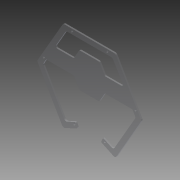
# Autodesk Inventor part: Top Plat
Saved by Autodesk Inventor 2015 (Build 190159000, 159)
## iProperties
Created: 2016-10-14
Part Number: Top Plat
Material: Polycarbonate, Clear
Document SubType Name: Modeling
Designer: James Yelland
Density: 1.2 g/cm^3
Appearance: Polycarbonate - Clear
Author: James Yelland
Autodesk Inventor part; units mm, degrees
ref_plane "YZ Plane" through (0, 0, 0) normal (1, 0, 0) x (0, 1, 0)
ref_plane "XZ Plane" through (0, 0, 0) normal (0, 1, 0) x (-1, 0, 0)
ref_plane "XY Plane" through (0, 0, 0) normal (0, 0, 1) x (1, 0, 0)
sketch "Sketch1" plane through (0, 0, 0) normal (0, 1, 0) x (-1, 0, 0)
  circle A0 centre (30.6147, -73.9104) radius 1.6
  circle A1 centre (-30.6147, -73.9104) radius 1.6
  circle A2 centre (30.6147, -73.9104) radius 1.6
  circle A3 centre (-30.6147, -73.9104) radius 1.6
  line L0 (103.5566, -2.5) -> (54.8095, -86.9325)
  line L1 (-54.8095, -86.9325) -> (-103.5566, -2.5)
  line L2 (-103.5566, 2.5) -> (-53.9434, 88.4327)
  line L3 (-49.6132, 90.9327) -> (49.6132, 90.9327)
  line L4 (53.9434, 88.4327) -> (103.5566, 2.5)
  arc A4 (48.3297, -88.9468) -> (54.8095, -86.9325) centre (50.4794, -84.4325) ccw
  arc A5 (-54.8095, -86.9325) -> (-48.3297, -88.9468) centre (-50.4794, -84.4325) ccw
  arc A6 (-103.5566, 2.5) -> (-103.5566, -2.5) centre (-99.2265, 0) ccw
  arc A7 (-49.6132, 90.9327) -> (-53.9434, 88.4327) centre (-49.6132, 85.9327) ccw
  arc A8 (53.9434, 88.4327) -> (49.6132, 90.9327) centre (49.6132, 85.9327) ccw
  arc A9 (103.5566, -2.5) -> (103.5566, 2.5) centre (99.2265, 0) ccw
  arc A10 (-43.8396, 80.9325) -> (-48.1698, 78.4325) centre (-43.8396, 75.9325) ccw
  arc A11 (-92.0094, 2.5) -> (-92.0094, -2.5) centre (-87.6793, 0) ccw
  line L5 (32.3518, -70.2624) -> (44.2883, -75.9464)
  arc A12 (44.2883, -75.9464) -> (50.7681, -73.9321) centre (46.4379, -71.4321) ccw
  line L6 (32.3518, -70.2624) -> (29.6432, -68.9726)
  line L7 (26.9776, -69.9184) -> (24.398, -75.3356)
  arc A13 (29.6432, -68.9726) -> (26.9776, -69.9184) centre (28.7834, -70.7783) ccw
  arc A14 (24.398, -75.3356) -> (25.3439, -78.0012) centre (26.2038, -76.1955) ccw
  circle A15 centre (-30.6147, -73.9104) radius 1.6
  circle A16 centre (-30.6147, -73.9104) radius 1.6
  line L8 (-32.3518, -70.2624) -> (-44.2883, -75.9464)
  arc A17 (-50.7681, -73.9321) -> (-44.2883, -75.9464) centre (-46.4379, -71.4321) ccw
  line L9 (-32.3518, -70.2624) -> (-29.6432, -68.9726)
  line L10 (-26.9776, -69.9184) -> (-24.398, -75.3356)
  arc A18 (-26.9776, -69.9184) -> (-29.6432, -68.9726) centre (-28.7834, -70.7783) ccw
  arc A19 (-25.3439, -78.0012) -> (-24.398, -75.3356) centre (-26.2038, -76.1955) ccw
  line L11 (48.3297, -88.9468) -> (25.3439, -78.0012)
  line L12 (-25.3439, -78.0012) -> (-48.3297, -88.9468)
  arc A20 (48.1698, 78.4325) -> (43.8396, 80.9325) centre (43.8396, 75.9325) ccw
  arc A21 (92.0094, -2.5) -> (92.0094, 2.5) centre (87.6793, 0) ccw
  circle A22 centre (35.5991, 85.9437) radius 1.6
  circle A23 centre (-35.5945, 85.9327) radius 1.6
  circle A24 centre (92.2171, 12.1406) radius 1.6
  circle A25 centre (-92.2171, 12.1406) radius 1.6
  line L13 (-18.2679, -8.3495) -> (18.2679, -8.3495)
  line L14 (-92.0094, -2.5) -> (-50.7681, -73.9321)
  line L15 (50.7681, -73.9321) -> (92.0094, -2.5)
  line L16 (59.1367, 11.2915) -> (33.0718, 11.2915)
  line L17 (59.1367, 11.2915) -> (85.2016, 11.2915)
  line L18 (53.75, 35.5415) -> (53.75, 17.0415)
  line L19 (53.75, 17.0415) -> (41.25, 17.0415)
  line L20 (41.25, 17.0415) -> (41.25, 35.5415)
  line L21 (41.25, 35.5415) -> (53.75, 35.5415)
  line L22 (53.75, 35.5415) -> (41.25, 17.0415) construction
  line L23 (53.75, 17.0415) -> (41.25, 35.5415) construction
  line L24 (71.75, 35.5415) -> (71.75, 17.0415)
  line L25 (71.75, 17.0415) -> (59.25, 17.0415)
  line L26 (59.25, 17.0415) -> (59.25, 35.5415)
  line L27 (59.25, 35.5415) -> (71.75, 35.5415)
  line L28 (71.75, 35.5415) -> (59.25, 17.0415) construction
  line L29 (71.75, 17.0415) -> (59.25, 35.5415) construction
  line L30 (92.0094, 2.5) -> (87.7997, 9.7915)
  line L31 (30.4737, 9.7915) -> (20.866, -6.8495)
  line L32 (-59.1367, 11.2915) -> (-33.0718, 11.2915)
  line L33 (-59.1367, 11.2915) -> (-85.2016, 11.2915)
  line L34 (-92.0094, 2.5) -> (-87.7997, 9.7915)
  line L35 (-30.4737, 9.7915) -> (-20.866, -6.8495)
  arc A26 (87.7997, 9.7915) -> (85.2016, 11.2915) centre (85.2016, 8.2915) ccw
  arc A27 (33.0718, 11.2915) -> (30.4737, 9.7915) centre (33.0718, 8.2915) ccw
  arc A28 (64.417, 41.2915) -> (67.0151, 45.7915) centre (64.417, 44.2915) ccw
  arc A29 (30.4737, 42.7915) -> (33.0718, 41.2915) centre (33.0718, 44.2915) ccw
  arc A30 (18.2679, -8.3495) -> (20.866, -6.8495) centre (18.2679, -5.3495) ccw
  arc A31 (-20.866, -6.8495) -> (-18.2679, -8.3495) centre (-18.2679, -5.3495) ccw
  arc A32 (-30.4737, 9.7915) -> (-33.0718, 11.2915) centre (-33.0718, 8.2915) ccw
  arc A33 (-33.0718, 41.2915) -> (-30.4737, 42.7915) centre (-33.0718, 44.2915) ccw
  arc A34 (-18.2679, 60.9325) -> (-20.866, 59.4325) centre (-18.2679, 57.9325) ccw
  arc A35 (20.866, 59.4325) -> (18.2679, 60.9325) centre (18.2679, 57.9325) ccw
  arc A36 (-67.0151, 45.7915) -> (-64.417, 41.2915) centre (-64.417, 44.2915) ccw
  arc A37 (-85.2016, 11.2915) -> (-87.7997, 9.7915) centre (-85.2016, 8.2915) ccw
  line L36 (43.8396, 80.9325) -> (-43.8396, 80.9325)
  line L37 (-48.1698, 78.4325) -> (-67.0151, 45.7915)
  line L38 (-64.417, 41.2915) -> (-33.0718, 41.2915)
  line L39 (-30.4737, 42.7915) -> (-20.866, 59.4325)
  line L40 (-18.2679, 60.9325) -> (18.2679, 60.9325)
  line L41 (20.866, 59.4325) -> (30.4737, 42.7915)
  line L42 (33.0718, 41.2915) -> (64.417, 41.2915)
  line L43 (67.0151, 45.7915) -> (48.1698, 78.4325)
  point P0 (105, 0)
  point P1 (52.5, -90.9327)
  point P2 (-105, 0)
  point P3 (-52.5, 90.9327)
  point P4 (52.5, 90.9327)
  point P5 (-93.4528, 0)
  point P6 (-46.7264, 80.9325)
  point P7 (46.7264, 80.9325)
  point P8 (93.4528, 0)
  point P9 (-5, -80.9325)
  point P10 (5, -80.9325)
  point P11 (69.6132, 41.2915)
  point P12 (86.9337, 11.2915)
  point P13 (-69.6132, 41.2915)
  point P14 (-86.9337, 11.2915)
  dimension "d148" = 5
  dimension "d150" = 2
  dimension "d199" = 5
  dimension "d231" = 18.5
  dimension "d232" = 12.5
  dimension "d234" = 18.5
  dimension "d235" = 12.5
  dimension "d236" = 3
  constraints: 88 end point, 57 point on circle, 38 centre point, 15 point on line, 12 equal radius, 12 tangent, 9 parallel, 3 coincident, 2 perpendicular, 1 horizontal, 1 vertical
  measures "d148" radius of A12
  measures "d150" radius of A13
  measures "d199" radius of A20
  measures "d231" distance of L18.start L18.end
  measures "d232" distance of L18.end L19.end
  measures "d234" distance of L24.start L24.end
  measures "d235" distance of L24.end L25.end
  measures "d236" radius of A26
extrude "Extrusion2" add sketch "Sketch1" along normal blind 3 contours L0 A4 L11 A14 L7 A13 L6 L5 A12 L15 A21 L30 A26 L17 L16 A27 L31 A30 L13 A31 L35 A32 L32 L33 A37 L34 A11 L14 A17 L8 L9 A18 L10 A19 L12 A5 L1 A6 L2 A7 L3 A8 L4 A9 | L18 L19 L20 L21 | L24 L25 L26 L27
body "Solid2"
